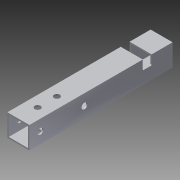
# Autodesk Inventor part: Camera Traffic Light Mount
Saved by Autodesk Inventor 2013 (Build 170138000, 138)
## iProperties
Created: 2013-01-24
Part Number: Camera Traffic Light Mount
Material: Acetal Resin, White
Document SubType Name: Modeling
Designer: actoennies
Density: 1.425 g/cm^3
Mass: 34.5638 g
Surface Area: 310.297 cm^2
Volume: 24.2553 cm^3
Author: actoennies
Autodesk Inventor part; units mm, degrees
ref_plane "YZ Plane" through (0, 0, 0) normal (1, 0, 0) x (0, 1, 0)
ref_plane "XZ Plane" through (0, 0, 0) normal (0, 1, 0) x (-1, 0, 0)
ref_plane "XY Plane" through (0, 0, 0) normal (0, 0, 1) x (1, 0, 0)
sketch "Sketch1" plane through (0, 0, 0) normal (0, 0, 1) x (1, 0, 0)
  line L0 (0, 0) -> (25.4, 0)
  line L1 (25.4, 0) -> (25.4, 25.4)
  line L2 (25.4, 25.4) -> (0, 25.4)
  line L3 (0, 25.4) -> (0, 0)
  line L4 (1.5875, 1.5875) -> (23.8125, 1.5875)
  line L5 (23.8125, 1.5875) -> (23.8125, 23.8125)
  line L6 (23.8125, 23.8125) -> (1.5875, 23.8125)
  line L7 (1.5875, 23.8125) -> (1.5875, 1.5875)
  dimension "d0" = 25.4
  dimension "d1" = 25.4
  dimension "d2" = 1.5875
  constraints: 16 end point, 4 parallel, 2 perpendicular, 1 horizontal, 3 other
  measures "d0" distance of L2.end L1.end
  measures "d1" distance of L2.end L0.start
  measures "d2" distance between parallel lines of L3 L7
extrude "Extrusion1" add sketch "Sketch1" along normal blind 165.1
sketch "Sketch2" plane through (0, 0, 0) normal (-1, 0, 0) x (0, 0, 1)
  arc A0 (33.3863, 14.478) -> (34.4023, 15.494) centre (33.3863, 15.494) ccw projected
  line L0 (34.4023, 15.494) -> (34.4023, 25.4) projected
  line L1 (34.4023, 25.4) -> (24.2423, 25.4) projected
  line L2 (24.2423, 25.4) -> (24.2423, 15.494) projected
  arc A1 (24.2423, 15.494) -> (25.2583, 14.478) centre (25.2583, 15.494) ccw projected
  line L3 (25.2583, 14.478) -> (33.3863, 14.478) projected
  circle A2 centre (29.3223, 19.05) radius 4.0005 projected
extrude "Extrusion2" cut sketch "Sketch2" against normal blind 25.4 contours L3 A1 L2 L1 L0 A0 | A2
sketch "Sketch3" plane through (0, 0, 0) normal (0, -1, 0) x (1, 0, 0)
  circle A0 centre (12.7, 142.875) radius 3.3782 projected
  circle A1 centre (12.7, 120.65) radius 3.3782 projected
extrude "Extrusion3" cut sketch "Sketch3" against normal blind 25.4
sketch "Sketch4" plane through (0, 0, 0) normal (-1, 0, 0) x (0, 0, 1)
  circle A0 centre (152.4, 12.7) radius 3.3782 projected
  circle A1 centre (101.6, 12.7) radius 3.3782 projected
extrude "Extrusion4" cut sketch "Sketch4" against normal blind 25.4
body "Solid1"
